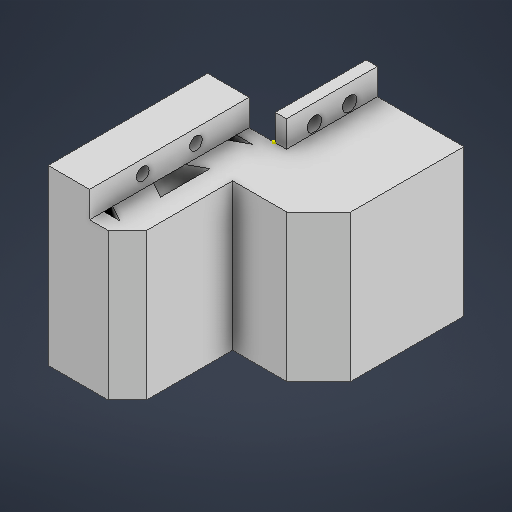
# Autodesk Inventor part: servo  holder
Saved by Autodesk Inventor 2026.1 (Build 301233000, 233)
## iProperties
Created: 2026-03-18
Part Number: servo  holder
Material: Generic
Document SubType Name: Modeling
Designer: ba2032
Density: 1 g/cm^3
Appearance: Default
Author: ba2032
Autodesk Inventor part; units mm, degrees
ref_plane "YZ Plane" through (0, 0, 0) normal (1, 0, 0) x (0, 1, 0)
ref_plane "XZ Plane" through (0, 0, 0) normal (0, 1, 0) x (-1, 0, 0)
ref_plane "XY Plane" through (0, 0, 0) normal (0, 0, 1) x (1, 0, 0)
sketch "Sketch1" plane through (0, 0, 0) normal (1, 0, 0) x (0, 1, 0)
  point P0 (0, 0)
sketch "Sketch2" plane through (0, 0, 0) normal (1, 0, 0) x (0, 1, 0)
  line L0 (0, 0) -> (0, -28.5)
  line L1 (0, -28.5) -> (46, -28.5)
  line L2 (46, -28.5) -> (46, 0)
  line L3 (46, 0) -> (0, 0)
  dimension "d0" = 28.5
  dimension "d1" = 46
  constraints: 8 end point, 2 parallel, 1 perpendicular, 1 vertical
  measures "d0" distance of L0.start L0.end
  measures "d1" distance of L1.end L0.end
sketch "Sketch3" plane through (0, 0, 0) normal (1, 0, 0) x (0, 1, 0)
  line L0 (2.5, -2.5) -> (2.5, -26)
  line L1 (2.5, -26) -> (43.5, -26)
  line L2 (43.5, -26) -> (43.5, -2.5)
  line L3 (43.5, -2.5) -> (2.5, -2.5)
  dimension "d6" = 23.5
  dimension "d7" = 41
  constraints: 8 end point, 2 parallel, 1 perpendicular, 1 vertical
  measures "d6" distance of L0.start L0.end
  measures "d7" distance of L1.end L0.end
extrude "Extrusion1" add sketch "Sketch2" along normal blind 30.6
extrude "Extrusion2" cut sketch "Sketch3" along normal blind 28.1
sketch "Sketch4" plane through (0, 0, -28.5) normal (0, 0, -1) x (-1, 0, 0)
  line L0 (0, 0) -> (0, -8.25)
  line L1 (0, -8.25) -> (-3.5, -8.25)
  line L2 (-3.5, -8.25) -> (-3.5, 0)
  line L3 (-3.5, 0) -> (0, 0)
  line L4 (0, 0) -> (0, 46) projected
  line L5 (0, 46) -> (0, 54.25)
  line L6 (0, 54.25) -> (-3.5, 54.25)
  line L7 (-3.5, 54.25) -> (-3.5, 46)
  line L8 (-3.5, 46) -> (0, 46)
  dimension "d10" = 8.25
  dimension "d11" = 3.5
  dimension "d16" = 8.25
  dimension "d17" = 3.5
  constraints: 16 end point, 4 parallel, 2 perpendicular, 1 collinear, 1 vertical
  measures "d10" distance of L0.start L0.end
  measures "d11" distance of L0.end L1.end
  measures "d16" distance of L4.end L5.end
  measures "d17" distance of L6.end L5.end
extrude "Extrusion3" add sketch "Sketch4" against normal blind 28.5 contours L0 L1 L2 L3
extrude "Extrusion4" add sketch "Sketch4" against normal blind 28.5 contours L8 L7 L6 L5
sketch "Sketch5" plane through (3.5, 46, -28.5) normal (1, 0, 0) x (0, 0, -1)
  circle A0 centre (-8.75, -48.25) radius 2.25
  circle A1 centre (-19.75, -48.25) radius 2.25
  circle A2 centre (-8.75, 2.5) radius 2.25
  circle A3 centre (-19.75, 2.5) radius 2.25
  point P0 (-28.5, -46)
  dimension "d25" = 4.5
  dimension "d26" = 4.5
  dimension "d27" = 4.5
  dimension "d28" = 4.5
  constraints: 4 centre point
  measures "d25" diameter of A0
  measures "d26" diameter of A1
  measures "d27" diameter of A2
  measures "d28" diameter of A3
extrude "Extrusion5" cut sketch "Sketch5" against normal blind 4.5
sketch "Sketch6" plane through (30.6, 0, -28.5) normal (0, -1, 0) x (1, 0, 0)
  line L0 (-2.5, 2.5) -> (-2.5, 26) projected
  line L1 (-2.5, 10.25) -> (-2.5, 18.25)
  line L2 (-2.5, 18.25) -> (-10.5, 18.25)
  line L3 (-10.5, 18.25) -> (-10.5, 10.25)
  line L4 (-10.5, 10.25) -> (-2.5, 10.25)
  point P0 (-30.6, 28.5)
  dimension "d29" = 8
  dimension "d30" = 8
  constraints: 8 end point, 2 parallel, 2 point on line, 1 perpendicular
  measures "d29" distance of L1.start L1.end
  measures "d30" distance of L2.end L1.end
extrude "Extrusion6" cut sketch "Sketch6" against normal blind 2.5
sketch "Sketch7" plane through (30.6, 0, 0) normal (0, 0, 1) x (1, 0, 0)
  line L0 (-30.6, 46) -> (-30.6, 0)
  line L1 (-30.6, 0) -> (-26.1, 0)
  line L2 (-26.1, 0) -> (-26.1, 46)
  line L3 (-26.1, 46) -> (-30.6, 46)
  dimension "d33" = 4.5
  constraints: 8 end point, 2 parallel, 1 perpendicular, 1 vertical
  measures "d33" distance of L1.end L0.end
extrude "Extrusion7" add sketch "Sketch7" along normal blind 50
sketch "Sketch8" plane through (0, 0, 0) normal (-1, 0, 0) x (0, 0, 1)
  line L0 (0, 46) -> (0, 0) projected
  line L1 (0, 0) -> (50, 0) projected
  line L2 (0, 0) -> (50, 0)
  line L3 (50, 0) -> (50, 46)
  line L4 (50, 46) -> (0, 46)
  line L5 (0, 46) -> (0, 0)
  constraints: 8 end point, 3 equal length, 1 perpendicular
extrude "Extrusion8" add sketch "Sketch8" along normal blind 21.2
sketch "Sketch9" plane through (30.6, 0, 0) normal (0, 0, 1) x (1, 0, 0)
  line L0 (-26.1, 0) -> (0, 0) projected
  line L1 (0, 46) -> (0, 0) projected
  line L2 (-26.1, 0) -> (0, 0)
  line L3 (0, 0) -> (0, 46)
  line L4 (0, 46) -> (-26.1, 46)
  line L5 (-26.1, 46) -> (-26.1, 0)
  point P0 (-30.6, 0)
  constraints: 8 end point, 2 parallel, 2 perpendicular
extrude "Extrusion9" add sketch "Sketch9" along normal blind 50
chamfer "Chamfer1" distance 33 angle 45 1 edges at (30.6, 23, 50)
sketch "Sketch10" plane through (3.5, 46, -28.5) normal (0, 1, 0) x (1, 0, 0)
  point P0 (-3.5, -28.5)
sketch "Sketch11" plane through (3.5, 46, -28.5) normal (0, 1, 0) x (1, 0, 0)
  line L0 (-3.5, -28.5) -> (-24.7, -28.5) projected
  line L1 (-20.7, -32.5) -> (-6.7, -32.5)
  line L2 (-20.7, -32.5) -> (-6.7, -32.5) construction
  line L3 (-6.7, -32.5) -> (-20.7, -40.246)
  line L4 (-20.7, -40.246) -> (-20.7, -32.5)
  line L5 (-5.9, -78.5) -> (-24.7, -78.5) projected
  line L6 (-20.7, -74.038) -> (-6.7, -74.038)
  line L7 (-20.7, -74.038) -> (-6.7, -74.038) construction
  line L8 (-6.7, -74.038) -> (-20.7, -66.292)
  line L9 (-20.7, -66.292) -> (-20.7, -74.038)
  line L10 (-6.7, -53.5) -> (9.3, -53.5) construction
  line L11 (-20.7, -53.5) -> (-6.7, -45.754)
  line L12 (-20.7, -53.5) -> (-6.7, -61.246)
  line L13 (-6.7, -61.246) -> (-6.7, -45.754)
  line L14 (-5.9, -78.5) -> (27.1, -45.5) projected
  line L15 (0.124, -72.476) -> (0.124, -45.5)
  line L16 (0.124, -45.5) -> (27.1, -45.5)
  dimension "d45" = 14
  dimension "d46" = 0
  dimension "d47" = 16
  dimension "d49" = 14
  dimension "d50" = 0
  dimension "d51" = 16
  dimension "d59" = 16
  dimension "d60" = 16
  constraints: 28 end point, 5 horizontal, 3 perpendicular, 2 collinear, 2 point on line, 2 vertical
  measures "d45" distance of L1.start L1.end
  measures "d46" distance between parallel lines of L1 L2
  measures "d47" distance of L1.end L3.end
  measures "d49" distance of L6.start L6.end
  measures "d50" distance between parallel lines of L6 L7
  measures "d51" distance of L6.end L8.end
  measures "d59" distance of L11.start L11.end
  measures "d60" distance of L11.start L12.end
extrude "Extrusion10" cut sketch "Sketch11" against normal blind 46
chamfer "Chamfer2" distance 10 angle 45 1 edges at (30.6, 23, 17)
sketch "Sketch12" plane through (-21.2, 0, 0) normal (-1, 0, 0) x (0, 0, 1)
  line L0 (-28.5, 46) -> (7, 46) projected
  line L1 (-28.5, 54.25) -> (0, 54.25) projected
  line L2 (0, 46) -> (0, 54.25)
  line L3 (0, 54.25) -> (50, 54.25)
  line L4 (50, 54.25) -> (50, 46)
  line L5 (50, 46) -> (0, 46)
  point P0 (0, 0)
  constraints: 8 end point, 2 parallel, 1 perpendicular, 1 point on line, 1 vertical
extrude "Extrusion11" add sketch "Sketch12" against normal blind 13
sketch "Sketch13" plane through (-8.2, 0, 0) normal (1, 0, 0) x (0, 0, -1)
  circle A0 centre (-16.6667, 50.125) radius 2
  circle A1 centre (-33.333, 50.125) radius 2
  point P0 (0, 0)
  dimension "d70" = 4
  dimension "d71" = 4
  constraints: 2 centre point
  measures "d70" diameter of A0
  measures "d71" diameter of A1
extrude "Extrusion12" cut sketch "Sketch13" against normal blind 13
equation "\"d23\" = d28"
body "Solid1"
